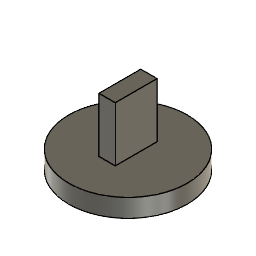
support-potent-aero-petit (Autodesk Fusion 360 design; units mm, degrees)
Autodesk Fusion 360 part; units mm, degrees
sketch "Esquisse1" plane through (0, 0, 0) normal (0, 0, 1) x (1, 0, 0)
  circle A0 centre (0, 0) radius 3.25
  dimension "d1" = 6.5
  constraint coincident A0.centre origin
  measures "d1" diameter of A0
extrude "Extrusion1" add sketch "Esquisse1" along normal blind 1
sketch "Esquisse2" plane through (0, 0, 1) normal (0, 0, 1) x (-1, 0, 0)
  circle A0 centre (0, 0) radius 3.25
  line L0 (-0.45, 1.15) -> (0.45, 1.15)
  line L1 (0.45, 1.15) -> (0.45, -1.15)
  line L2 (0.45, -1.15) -> (-0.45, -1.15)
  line L3 (-0.45, -1.15) -> (-0.45, 1.15)
  line L4 (-0.45, 1.15) -> (0.45, -1.15) construction
  line L5 (0.45, 1.15) -> (-0.45, -1.15) construction
  dimension "d4" = 0.9
  dimension "d5" = 2.3
  constraint horizontal L0
  constraint perpendicular L0 L1
  constraint parallel L0 L2
  constraint parallel L1 L3
  constraint coincident L4 A0.centre
  constraint coincident L5 A0.centre
  constraint coincident A0.centre origin
  measures "d4" distance of L1.end L2.end
  measures "d5" distance of L0.end L1.end
extrude "Extrusion2" add sketch "Esquisse2" along normal blind 3 contours L0 L1 L2 L3
